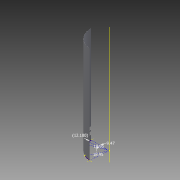
# Autodesk Inventor part: EDM Middle Shield Part 4
Saved by Autodesk Inventor 2015 (Build 190159000, 159)
## iProperties
Created: 2014-06-18
Part Number: EDM Middle Shield Part 4
Material: Generic
Document SubType Name: Modeling
Designer: Aki
Density: 1 g/cm^3
Appearance: Default
Author: Aki
Autodesk Inventor part; units mm, degrees
ref_plane "YZ Plane" through (0, 0, 0) normal (1, 0, 0) x (0, 1, 0)
ref_plane "XZ Plane" through (0, 0, 0) normal (0, 1, 0) x (-1, 0, 0)
sketch "Sketch1" plane through (0, 0, 0) normal (0, 1, 0) x (-1, 0, 0)
  arc A0 (307.34, 0) -> (25.3968, 306.2889) centre (0, 0) ccw
  line L0 (0, 0) -> (25.3968, 306.2889) construction
  line L1 (0, 0) -> (307.34, 0) construction
  arc A1 (306.07, 0) -> (25.2919, 305.0232) centre (0, 0) ccw
  line L2 (0, 0) -> (25.2919, 305.0232) construction
  line L3 (0, 0) -> (306.07, 0) construction
  line L4 (306.07, 0) -> (307.34, 0)
  line L5 (25.2919, 305.0232) -> (25.3968, 306.2889)
  dimension "d0" = 307.34
  dimension "d1" = 85.26
  dimension "d2" = 306.07
  dimension "d3" = 85.26
  constraints: 12 end point, 4 point on circle, 2 centre point, 2 coincident, 1 collinear
  measures "d0" radius of A0
  measures "d1" angle of L1 L0
  measures "d2" radius of A1
  measures "d3" angle of L3 L2
extrude "Extrusion1" add sketch "Sketch1" along normal blind 1625.6
sketch "Sketch2" plane through (0, 0, 0) normal (0, 1, 0) x (-1, 0, 0)
  arc A0 (307.34, 0) -> (303.1515, 50.567) centre (0, 0) ccw
  line L0 (0, 0) -> (303.1515, 50.567) construction
  line L1 (0, 0) -> (307.34, 0) construction
  arc A1 (307.34, 0) -> (290.6829, 99.8065) centre (0, 0) ccw
  line L2 (0, 0) -> (290.6829, 99.8065) construction
  line L3 (0, 0) -> (307.34, 0) construction
  arc A2 (123.4855, 281.4413) -> (25.3968, 306.2889) centre (0, 0) ccw
  line L4 (0, 0) -> (123.4855, 281.4413) construction
  line L5 (0, 0) -> (25.3968, 306.2889) construction
  dimension "d6" = 307.34
  dimension "d7" = 9.47
  dimension "d14" = 18.95
  dimension "d15" = 18.95
  constraints: 12 end point, 6 point on circle, 3 centre point, 3 coincident
  measures "d6" radius of A0
  measures "d7" angle of L1 L0
  measures "d14" angle of L3 L2
  measures "d15" angle of L4 L5
ref_plane "Work Plane1" through (-303.1515, 0, 50.567) normal (-0.9863719, 0, 0.1645312) x (0, -1, 0)
sketch "Sketch3" plane through (-303.1515, 0, 50.567) normal (-0.9863719, 0, 0.1645312) x (0, -1, 0)
  circle A0 centre (-103.1875, 0) radius 25.4
  line L0 (0, 297.9362) -> (0, -50.567) projected
  line L1 (0, -50.3581) -> (-1625.6, -50.3581) projected
  line L2 (-128.5875, 0) -> (-77.7875, 0)
  line L3 (-77.7875, 0) -> (-77.7875, -50.3581)
  line L4 (-77.7875, -50.3581) -> (-128.5875, -50.3581)
  line L5 (-128.5875, -50.3581) -> (-128.5875, 0)
  circle A1 centre (-176.2125, 0) radius 25.4
  line L6 (-201.6125, 0) -> (-150.8125, 0)
  line L7 (-150.8125, 0) -> (-150.8125, -50.3581)
  line L8 (-150.8125, -50.3581) -> (-201.6125, -50.3581)
  line L9 (-201.6125, -50.3581) -> (-201.6125, 0)
  point P0 (0, 0)
  dimension "d8" = 50.8
  dimension "d10" = 50.8
  dimension "d9" = 103.1875
  dimension "d11" = 176.2125
  constraints: 16 end point, 4 parallel, 2 horizontal, 2 horizontal alignment, 2 perpendicular, 2 point on line, 4 other
  measures "d9" distance from line of L0 point (-103.188, 0)
  measures "d11" distance from line of L0 point (-176.213, 0)
extrude "Extrusion2" cut sketch "Sketch3" against normal blind 25.4
body "Solid1"
